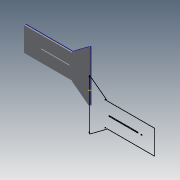
# Autodesk Inventor part: sideplate
Saved by Autodesk Inventor 2015 (Build 190159000, 159)
## iProperties
Created: 2014-08-31
Part Number: sideplate
Material: Generic
Document SubType Name: Modeling
Designer: shohei
Density: 1 g/cm^3
Appearance: Default
Mass: 5703.68 g
Surface Area: 6418.8 cm^2
Volume: 5703.68 cm^3
Author: shohei
Autodesk Inventor part; units mm, degrees
ref_plane "YZ Plane" through (0, 0, 0) normal (1, 0, 0) x (0, 1, 0)
ref_plane "XZ Plane" through (0, 0, 0) normal (0, 1, 0) x (-1, 0, 0)
ref_plane "XY Plane" through (0, 0, 0) normal (0, 0, 1) x (1, 0, 0)
sketch "Block1" plane through (0, 0, 0) normal (0, 0, 1) x (1, 0, 0)
  line L0 (-221.2939, -300.22) -> (-810.22, -300.22)
  line L1 (-810.22, -300.22) -> (-810.22, 0.22)
  line L2 (-810.22, 0.22) -> (-221.2939, 0.22)
  line L3 (-221.2939, 0.22) -> (-10.7624, 210.7619)
  arc A0 (0.22, 215.2184) -> (-10.7624, 210.7619) centre (0, 200) ccw
  line L4 (0.22, 215.2184) -> (0.22, -515.2184)
  arc A1 (-10.7624, -510.7619) -> (0.22, -515.2184) centre (0, -500) ccw
  line L5 (-10.7624, -510.7619) -> (-221.2939, -300.22)
  line L6 (-600.3559, -155.3081) -> (-250.3559, -155.3081)
  arc A2 (-250.3559, -155.3081) -> (-250, -144.68) centre (-250, -150) ccw
  line L7 (-250, -144.68) -> (-599.9854, -144.68)
  line L8 (-599.9854, -144.68) -> (-600.0274, -144.6801)
  arc A3 (-600.0274, -144.6801) -> (-600.3559, -155.3081) centre (-600, -150) ccw
  circle A4 centre (-650, -150) radius 5.22
  point P0 (-340.1003, -149.6438)
sketch "Block2" plane through (0, 0, 0) normal (0, 0, 1) x (1, 0, 0)
  line L0 (-810.22, -300.22) -> (-810.22, 0.22)
  line L1 (-810.22, 0.22) -> (-215.2184, 0.22)
  arc A0 (-208.9704, 12.2955) -> (-215.2184, 0.22) centre (-200, 0) ccw
  line L2 (-208.9704, 12.2955) -> (-9.1321, 162.176)
  arc A1 (0.22, 165.2184) -> (-9.1321, 162.176) centre (0, 150) ccw
  line L3 (0.22, 165.2184) -> (0.22, -465.2184)
  arc A2 (-9.132, -462.176) -> (0.22, -465.2184) centre (0, -450) ccw
  line L4 (-9.132, -462.176) -> (-209.25, -312.0866)
  arc A3 (-215.2184, -300.22) -> (-209.25, -312.0866) centre (-200, -300) ccw
  line L5 (-215.2184, -300.22) -> (-810.22, -300.22)
  line L6 (-600.3526, -155.2081) -> (-250.3526, -155.2081)
  arc A4 (-250.3526, -155.2081) -> (-250, -144.78) centre (-250, -150) ccw
  line L7 (-250, -144.78) -> (-599.9853, -144.78)
  line L8 (-599.9853, -144.78) -> (-600.0271, -144.7801)
  arc A5 (-600.0271, -144.7801) -> (-600.3526, -155.2081) centre (-600, -150) ccw
  circle A6 centre (-650, -150) radius 5.22
  point P0 (-319.1116, -149.6914)
sketch "Sketch1" plane through (0, 0, 0) normal (0, 1, 0) x (-1, 0, 0)
  line L0 (215, 0) -> (810, 0)
  line L1 (810, 0) -> (810, 300)
  line L2 (810, 300) -> (215, 300)
  line L3 (0, 300) -> (0, 0)
  line L4 (-166.7515, 0) -> (998.9689, 0) projected
  line L5 (0, -579.8647) -> (0, 1964.869) projected
  line L6 (998.9689, 0) -> (-166.7515, 0) projected
  arc A0 (9, 462) -> (0, 465) centre (0, 450) ccw
  arc A1 (0, -165) -> (9.0001, -162) centre (0, -150) ccw
  arc A2 (215, 300) -> (209.1171, 311.9113) centre (200, 300) ccw
  arc A3 (208.8396, -12.1186) -> (215, 0) centre (200, 0) ccw
  line L7 (209.1171, 311.9113) -> (9, 462)
  line L8 (208.8396, -12.1186) -> (9.0001, -162)
  line L9 (0, 465) -> (0, 300)
  line L10 (0, -165) -> (0, 0)
  arc A4 (599.9852, 145) -> (604.9434, 150.7503) centre (600, 150) ccw
  circle A5 centre (650, 150) radius 5
  arc A6 (599.9852, 145) -> (599.655, 154.9881) centre (600, 150) ccw
  line L11 (599.9852, 145) -> (600.0264, 145.0001)
  arc A7 (599.9852, 145) -> (599.655, 154.9881) centre (600, 150) ccw
  arc A8 (250.345, 154.9881) -> (250, 145) centre (250, 150) ccw
  line L12 (600.345, 154.9881) -> (250, 154.9881)
  line L13 (599.9852, 145) -> (250, 145)
  arc A9 (9.132, 462.176) -> (-0.22, 465.2184) centre (0, 450) ccw
  line L14 (-0.22, 465.2184) -> (-0.22, 300)
  line L15 (-0.22, 300) -> (-0.22, 0)
  line L16 (-0.22, 0) -> (-0.22, -165.2184)
  arc A10 (-0.22, -165.2184) -> (9.1321, -162.176) centre (0, -150) ccw
  line L17 (9.1321, -162.176) -> (225.0709, -0.22)
  line L18 (225.0709, -0.22) -> (810.22, -0.22)
  line L19 (810.22, -0.22) -> (810.22, 300.22)
  line L20 (810.22, 300.22) -> (225.072, 300.22)
  line L21 (225.072, 300.22) -> (9.132, 462.176)
  point P0 (400.5629, 131.6754)
  point P1 (595.0566, 150.7503)
  dimension "d25" = 810
  dimension "d26" = 30
  dimension "d27" = 30
  dimension "d28" = 150
  dimension "d29" = 150
  dimension "d30" = 30
  dimension "d31" = 30
  dimension "d32" = 200
  dimension "d33" = 200
  dimension "d35" = 10
  dimension "d36" = 10
  dimension "d39" = 50
  dimension "d42" = 300
  dimension "d43" = 300
  dimension "d44" = 150
  dimension "d46" = 10
  dimension "d47" = 150
  dimension "d48" = 250
  dimension "d49" = 350
  dimension "d50" = 0.22
  constraints: 38 end point, 26 point on circle, 11 centre point, 10 point on line, 4 collinear, 4 parallel, 3 tangent, 2 coincident, 2 horizontal, 2 perpendicular, 1 concentric, 9 other
  measures "d25" distance of L1.end L3.start
  measures "d26" diameter of A1
  measures "d27" diameter of A0
  measures "d28" distance from line of A0.centre L2
  measures "d29" distance from line of A1.centre L0
  measures "d30" diameter of A2
  measures "d31" diameter of A3
  measures "d32" distance from line of L5 A2.centre
  measures "d33" distance from line of L3 A3.centre
  measures "d35" diameter of A4
  measures "d36" diameter of A5
  measures "d39" distance of A5.centre A4.centre
  measures "d42" distance of L3.end L3.start
  measures "d43" distance of L0.end L1.end
  measures "d44" distance from line of L0 A4.centre
  measures "d46" diameter of A8
  measures "d47" distance from line of L4 A8.centre
  measures "d48" distance from line of L3 A8.centre
  measures "d49" distance of A8.centre A6.centre
  measures "d50" distance between parallel lines of L7 L21
extrude "Extrusion2" add sketch "Sketch1" along normal blind 20 contours L4 L3 L5 A0 L7 A2 L2 L1 L0 | A3 L8 A1 L5 L4 | L12 A6
sketch "Sketch5" plane through (0, 20, 0) normal (0, 1, 0) x (1, 0, 0)
  line L0 (-600.0264, -145.0001) -> (-599.9852, -145) projected
  line L1 (-599.9852, -145) -> (-250, -145) projected
  arc A0 (-250.345, -154.9881) -> (-250, -145) centre (-250, -150) ccw projected
  line L2 (-250.345, -154.9881) -> (-600.345, -154.9881) projected
  arc A1 (-600.0264, -145.0001) -> (-600.345, -154.9881) centre (-600, -150) ccw projected
  circle A2 centre (-650, -150) radius 5 projected
  line L3 (0, -465) -> (0, 165) projected
  arc A3 (0, 165) -> (-9.0001, 162) centre (0, 150) ccw projected
  line L4 (-9.0001, 162) -> (-208.8396, 12.1186) projected
  arc A4 (-208.8396, 12.1186) -> (-215, 0) centre (-200, 0) ccw projected
  line L5 (-215, 0) -> (-810, 0) projected
  line L6 (-810, 0) -> (-810, -300) projected
  line L7 (-810, -300) -> (-215, -300) projected
  arc A5 (-215, -300) -> (-209.1171, -311.9113) centre (-200, -300) ccw projected
  line L8 (-209.1171, -311.9113) -> (-9, -462) projected
  arc A6 (-9, -462) -> (0, -465) centre (0, -450) ccw projected
  point P0 (0, 0)
  constraints: 4 line through centre, 3 tangent, 1 perpendicular, 12 other
sketch "DXF" plane through (0, 0, 0) normal (0, 1, 0) x (-1, 0, 0)
  point P0 (0, 0)
equation "\"d50\" = Kerf"
equation "\"Kerf\" = 0.22"
body "Solid2"
